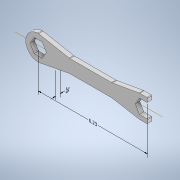
# Autodesk Inventor part: 3_4_inchWrenchV04
Saved by Autodesk Inventor 2020.3 (Build 243373000, 373)
## iProperties
Created: 2019-11-16
Part Number: 3_4_inchWrenchV04
Material: Generic
Document SubType Name: Modeling
Designer: steele
Density: 1 g/cm^3
Appearance: Default
Author: steele
Autodesk Inventor part; units mm, degrees
ref_plane "YZ Plane" through (0, 0, 0) normal (1, 0, 0) x (0, 1, 0)
ref_plane "XZ Plane" through (0, 0, 0) normal (0, 1, 0) x (-1, 0, 0)
ref_plane "XY Plane" through (0, 0, 0) normal (0, 0, 1) x (1, 0, 0)
sketch "Sketch2" plane through (0, 0, 0) normal (0, 0, 1) x (1, 0, 0)
  line L0 (-64.4682, 0) -> (-70.3341, -10.16)
  line L1 (-70.3341, -10.16) -> (-82.0659, -10.16)
  line L2 (-82.0659, -10.16) -> (-87.9318, 0)
  line L3 (-87.9318, 0) -> (-82.0659, 10.16)
  line L4 (-82.0659, 10.16) -> (-70.3341, 10.16)
  line L5 (-70.3341, 10.16) -> (-64.4682, 0)
  line L6 (-76.2, 0) -> (76.2, 0) construction
  line L7 (82.0659, -10.16) -> (70.3341, -10.16)
  line L8 (70.3341, -10.16) -> (64.4682, 0)
  line L9 (64.4682, 0) -> (70.3341, 10.16)
  line L10 (70.3341, 10.16) -> (82.0659, 10.16)
  line L11 (82.0659, 10.16) -> (82.4325, 9.525)
  line L12 (-132.627, 0) -> (135.7899, 0) projected
  line L13 (0, 0) -> (0, 37.2208) construction
  line L14 (0, 9.525) -> (30.7487, 9.525)
  line L15 (0, 9.525) -> (-30.7487, 9.525)
  circle A0 centre (-76.2, 0) radius 18.0818
  line L16 (-87.9318, 0) -> (-94.2818, 0) construction
  arc A1 (61.0244, 14.8673) -> (61.0244, -14.8673) centre (76.2, 0) ccw
  line L17 (87.9318, 0) -> (97.4446, 0) construction
  line L18 (87.9318, 0) -> (89.9839, -16.166) construction
  line L19 (30.7487, 9.525) -> (70.3341, 16.51)
  line L20 (-76.2, 18.0818) -> (-30.7487, 9.525)
  line L21 (70.3341, 10.16) -> (70.3341, 16.51) construction
  line L22 (82.0659, 10.16) -> (82.0659, 16.51)
  line L23 (82.0659, -10.16) -> (82.0659, -16.51)
  line L24 (0, -9.525) -> (30.7487, -9.525)
  line L25 (0, -9.525) -> (-30.7487, -9.525)
  line L26 (30.7487, -9.525) -> (70.3341, -16.51)
  line L27 (-76.2, -18.0818) -> (-30.7487, -9.525)
  line L28 (70.3341, 16.51) -> (82.0659, 16.51)
  line L29 (70.3341, -10.16) -> (70.3341, -16.51) construction
  line L30 (70.3341, -16.51) -> (82.0659, -16.51)
  point P0 (82.0659, 18.5801)
  point P1 (82.0659, -18.5801)
  dimension "centerToBoxEndWrench" = 76.2
  dimension "boltPrintedSize" = 20.32
  dimension "centerToOpenEndWrench" = 76.2
  dimension "d23" = 9.525
  dimension "d24" = 6.35
  dimension "d26" = 6.35
  constraints: 60 end point, 6 point on line, 5 horizontal, 5 symmetric about line, 4 point on circle, 4 vertical, 3 coincident, 3 collinear, 2 centre point, 2 perpendicular, 24 other
  measures "centerToBoxEndWrench" distance of L6.start L13.start
  measures "boltPrintedSize" distance between parallel lines of L1 L4
  measures "centerToOpenEndWrench" distance of L6.end L13.start
  measures "d23" distance between parallel lines of L14 L12
  measures "d24" distance of L16.end L2.end
  measures "d26" distance of L19.end L9.end
extrude "Extrusion2" add sketch "Sketch2" along normal mid plane 6.35 contours L12 A0 L27 L2 L1 L0 | L5 L4 L3 L12 A0 L20 | A0 L20 L15 L14 L19 A1 L12 | L12 A1 L26 L24 L25 L27 A0 | A1 L19 L28 L22 L10 L9 L12 | L12 L8 L7 L23 L30 L26 A1
fillet "Fillet1" radius 0.7937 4 edges at (82.0659, 16.51, 0) (82.0659, 10.16, 0) (82.0659, -10.16, 0) (82.0659, -16.51, 0)
fillet "Fillet2" radius 6.35 8 edges at (-30.7487, -9.525, 0) (30.7487, -9.525, 0) (70.3341, -16.51, 0) (-76.2, -18.0818, 0) (-76.2, 18.0818, 0) (-30.7487, 9.525, 0) (30.7487, 9.525, 0) (70.3341, 16.51, 0)
equation "\"centerToBoxEndWrench\" = 4 * boltSize"
equation "\"boltPrintedSize\" = boltSize + boltGap"
equation "\"centerToOpenEndWrench\" = 4 * boltSize"
equation "\"d23\" = 0.5 * boltSize"
equation "\"d24\" = minWallThickness"
equation "\"d26\" = minWallThickness"
equation "\"d27\" = minWallThickness"
equation "\"minWallThickness\" = 6.35"
equation "\"boltGap\" = 1.27"
equation "\"boltSize\" = 19.05"
body "Solid2"
